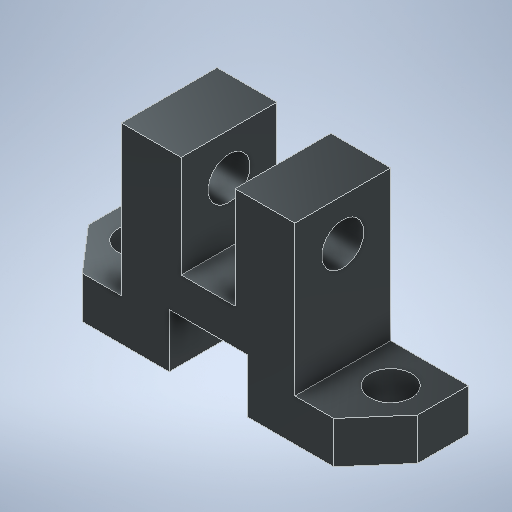
# Autodesk Inventor part: cad@26
Saved by Autodesk Inventor 2025.2 (Build 292293000, 293)
## iProperties
Created: 2025-03-15
Part Number: cad@26
Material: Iron, Cast
Document SubType Name: Modeling
Designer: spars
Density: 7.15 g/cm^3
Appearance: Iron Gray
Author: spars
Autodesk Inventor part; units mm, degrees
ref_plane "YZ Plane" through (0, 0, 0) normal (1, 0, 0) x (0, 1, 0)
ref_plane "XZ Plane" through (0, 0, 0) normal (0, 1, 0) x (-1, 0, 0)
ref_plane "XY Plane" through (0, 0, 0) normal (0, 0, 1) x (1, 0, 0)
sketch "Sketch1" plane through (0, 0, 0) normal (0, 0, 1) x (1, 0, 0)
  line L0 (-14.5, -16) -> (14.5, -16)
  line L1 (14.5, -16) -> (14.5, 16)
  line L2 (14.5, 16) -> (-14.5, 16)
  line L3 (-14.5, 16) -> (-14.5, -16)
  line L4 (-14.5, -16) -> (14.5, 16) construction
  line L5 (14.5, -16) -> (-14.5, 16) construction
  line L6 (-6.5, -16) -> (-6.5, -7)
  line L7 (6.5, -7) -> (6.5, -16)
  line L8 (-6.5, -7) -> (6.5, -7)
  line L9 (-4.5, -1) -> (4.5, -1)
  line L10 (-4.5, 16) -> (-4.5, -1)
  line L11 (4.5, 16) -> (4.5, -1)
  point P0 (0, 0)
  dimension "d0" = 29
  dimension "d1" = 32
  dimension "d8" = 9
  dimension "d9" = 8
  dimension "d10" = 8
  dimension "d11" = 9
  dimension "d12" = 17
  constraints: 24 end point, 5 perpendicular, 4 point on line, 2 midpoint, 2 parallel, 1 horizontal, 1 vertical
  measures "d0" distance of L2.end L1.end
  measures "d1" distance of L1.end L0.end
  measures "d8" distance of L6.start L6.end
  measures "d9" distance between parallel lines of L3 L6
  measures "d10" distance between parallel lines of L7 L1
  measures "d11" distance of L7.start L7.end
  measures "d12" distance between parallel lines of L9 L2
extrude "Extrusion1" add sketch "Sketch1" along normal blind 16 contours L3 L2 L10 L9 L11 L1 L0 L7 L8 L6
sketch "Sketch2" plane through (14.5, -16, 0) normal (1, 0, 0) x (0, 0, -1)
  line L0 (-16, 32) -> (-16, 0) projected
  line L1 (-16, 7) -> (0, 7)
  line L2 (0, 0) -> (-16, 0) projected
  line L3 (-16, 9) -> (-16, 0) projected
  line L4 (-16, 7) -> (-16, 0)
  line L5 (0, 0) -> (-16, 0) projected
  line L6 (-16, 0) -> (0, 0)
  line L7 (0, 0) -> (0, 7)
  line L8 (0, 0) -> (0, 9) projected
  point P0 (0, 16)
  dimension "d15" = 7
  constraints: 8 end point, 3 collinear, 1 horizontal, 1 point on line
  measures "d15" distance between parallel lines of L2 L1
extrude "Extrusion2" add sketch "Sketch2" along normal blind 13
sketch "Sketch3" plane through (-14.5, -16, 0) normal (-1, 0, 0) x (0, 0, 1)
  line L0 (0, 0) -> (16, 0) projected
  line L1 (0, 0) -> (0, 7) projected
  line L2 (0, 0) -> (0, 7)
  line L3 (16, 7) -> (0, 7) projected
  line L4 (0, 7) -> (16, 7)
  line L5 (16, 7) -> (16, 0)
  line L6 (16, 0) -> (0, 0)
  point P0 (0, 16)
  dimension "d18" = 7
  constraints: 8 end point, 2 collinear, 2 perpendicular
  measures "d18" distance of L0.start L1.end
extrude "Extrusion3" add sketch "Sketch3" along normal blind 13
sketch "Sketch4" plane through (-14.5, 16, 0) normal (-1, 0, 0) x (0, 0, 1)
  circle A0 centre (8, -7) radius 3.5
  line L0 (0, 0) -> (16, 0) projected
  line L1 (16, 0) -> (16, -25) projected
  line L2 (0, 0) -> (0, -25) projected
  point P0 (0, -16)
  dimension "d21" = 7
  dimension "d22" = 7
  dimension "d23" = 16
  dimension "d24" = 8
  constraints: 1 centre point
  measures "d21" diameter of A0
  measures "d22" distance from line of A0.centre L0
  measures "d23" distance between parallel lines of L1 L2
  measures "d24" distance from line of L2 A0.centre
extrude "Extrusion4" cut sketch "Sketch4" against normal through all
sketch "Sketch5" plane through (14.5, -9, 16) normal (0, 1, 0) x (1, 0, 0)
  line L0 (0, 0) -> (0, 16) projected
  line L1 (0, 0) -> (13, 0) projected
  line L2 (13, 16) -> (13, 0) projected
  line L3 (0, 16) -> (13, 16) projected
  line L4 (13, 16) -> (13, 6)
  line L5 (13, 0) -> (5.5, 0)
  line L6 (0, 0) -> (13, 0) projected
  line L7 (13, 16) -> (13, 0) projected
  line L8 (13, 0) -> (13, 6)
  circle A0 centre (6.5, 9.5) radius 3.5
  point P0 (-14.5, 16)
  dimension "d28" = 10
  dimension "d29" = 7.5
  dimension "d36" = 7
  constraints: 6 end point, 2 point on line, 1 centre point, 1 collinear
  measures "d28" distance of L2.start L4.end
  measures "d29" distance of L1.end L5.end
  measures "d36" diameter of A0
extrude "Extrusion5" cut sketch "Sketch5" against normal through all contours A0
sketch "Sketch6" plane through (14.5, -9, 16) normal (0, 1, 0) x (1, 0, 0)
  line L0 (-8, 0) -> (13, 0) projected
  line L1 (13, 0) -> (6.5, 0)
  line L2 (13, 0) -> (13, 7.5)
  line L3 (13, 0) -> (13, 16) projected
  line L4 (13, 7.5) -> (6.5, 0)
  point P0 (-14.5, 16)
  dimension "d39" = 6.5
  dimension "d40" = 7.5
  constraints: 6 end point, 2 point on line
  measures "d39" distance of L0.end L1.end
  measures "d40" distance of L0.end L2.end
extrude "Extrusion6" cut sketch "Sketch6" against normal through all
sketch "Sketch7" plane through (-14.5, -9, 16) normal (0, 1, 0) x (1, 0, 0)
  line L0 (8, 16) -> (-13, 16) projected
  line L1 (-13, 16) -> (-13, 0) projected
  circle A0 centre (-6.5, 9.5) radius 3.5
  line L2 (-13, 0) -> (-13, 7.5)
  line L3 (8, 0) -> (-13, 0) projected
  line L4 (-13, 0) -> (-6.5, 0)
  line L5 (-6.5, 0) -> (-13, 7.5)
  point P0 (14.5, 16)
  dimension "d44" = 7
  dimension "d46" = 7.5
  dimension "d47" = 6.5
  constraints: 6 end point, 2 point on line, 1 centre point
  measures "d44" diameter of A0
  measures "d46" distance of L1.end L2.end
  measures "d47" distance of L1.end L4.end
extrude "Extrusion7" cut sketch "Sketch7" against normal through all contours A0
sketch "Sketch8" plane through (-14.5, -9, 16) normal (0, 1, 0) x (1, 0, 0)
  line L0 (8, 0) -> (-13, 0) projected
  line L1 (-13, 0) -> (-6.5, 0)
  line L2 (-6.5, 0) -> (-13, 0)
  line L3 (-13, 0) -> (-13, 7.5)
  line L4 (-13, 16) -> (-13, 0) projected
  line L5 (-13, 7.5) -> (-6.5, 0)
  point P0 (14.5, 16)
  dimension "d50" = 6.5
  dimension "d51" = 7.5
  constraints: 8 end point, 2 point on line, 1 collinear
  measures "d50" distance of L0.end L1.end
  measures "d51" distance of L0.end L3.end
extrude "Extrusion8" cut sketch "Sketch8" against normal through all
body "Solid1"
